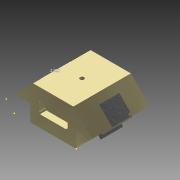
# Autodesk Inventor part: Correct middle piece Thursday 16
Saved by Autodesk Inventor 2015 (Build 190159000, 159)
## iProperties
Created: 2015-04-16
Part Number: Correct middle piece Thursday 16
Material: Generic
Document SubType Name: Modeling
Designer: Simrun
Density: 1 g/cm^3
Appearance: Gold - Metal
Author: Simrun
Autodesk Inventor part; units mm, degrees
sketch "Sketch1" plane through (0, 0, 0) normal (0, 0, 1) x (1, 0, 0)
  line L0 (0, 0) -> (171.45, 0)
  line L1 (171.45, 0) -> (171.45, 77.724)
  line L2 (171.45, 77.724) -> (0, 77.724)
  line L3 (0, 77.724) -> (0, 0)
  dimension "d0" = 171.45
  dimension "d1" = 77.724
  constraints: 8 end point, 2 parallel, 1 horizontal, 1 perpendicular
  measures "d0" distance of L2.end L1.end
  measures "d1" distance of L1.end L0.end
extrude "Extrusion1" add sketch "Sketch1" against normal blind 127
chamfer "Chamfer1" distance 41.275 angle 45 1 edges at (171.45, 77.724, -63.5)
chamfer "Chamfer2" distance 36.449 angle 45 1 edges at (171.45, 0, -63.5)
chamfer "Chamfer3" distance 41.275 angle 45 1 edges at (0, 77.724, -63.5)
chamfer "Chamfer4" distance 36.449 angle 45 1 edges at (0, 0, -63.5)
sketch "Sketch2" plane through (0, 0, 0) normal (0, 0, 1) x (1, 0, 0)
  point P0 (0, 0)
ref_plane "Work Plane1" through (0, 38.862, 0) normal (0, 1, 0) x (-1, 0, 0)
ref_plane "Work Plane4" through (85.725, 793.6029, -127) normal (1, 0, 0) x (0, 0, -1)
ref_plane "Work Plane2" through (130.175, 77.724, -127) normal (0.9980779, 0.0619722, 0) x (0, 0, 1)
ref_plane "Work Plane3" through (41.275, 77.724, -127) normal (0.9980779, -0.0619722, 0) x (0, 0, 1)
ref_plane "Work Plane5" through (171.45, 36.449, 0) normal (0, 1, 0) x (0, 0, -1)
ref_plane "Work Plane7" through (136.398, 36.449, 0) normal (1, 0, 0) x (0, 1, 0)
ref_plane "Work Plane6" through (171.45, 36.449, 0) normal (1, 0, 0) x (0, 1, 0)
sketch "Sketch3" plane through (136.398, 36.449, 0) normal (1, 0, 0) x (0, 1, 0)
  line L0 (-36.449, 0) -> (0, 0)
  line L1 (0, 0) -> (41.275, 0) projected
  arc A0 (-34.925, -22.225) -> (0, 0) centre (-33.1023, 13.4644) ccw
  line L2 (-34.925, -22.225) -> (-34.925, 0)
  dimension "d17" = 36.449
  constraints: 4 end point, 2 point on circle, 2 point on line, 1 centre point, 1 vertical
  measures "d17" distance of L0.start L0.end
extrude "Extrusion2" add sketch "Sketch3" along normal blind 34.925
sketch "Sketch4" plane through (171.323, 36.449, 0) normal (1, 0, 0) x (0, 0, -1)
  line L0 (0, -34.925) -> (0, 0)
  line L1 (0, -36.449) -> (0, 0) projected
  arc A0 (22.225, -34.925) -> (0, 0) centre (-13.4644, -33.1023) ccw
  line L2 (22.225, -34.925) -> (0, -34.925)
  line L3 (127, -36.449) -> (0, -36.449) projected
  constraints: 4 end point, 2 point on circle, 1 centre point, 1 collinear, 1 parallel
extrude "Extrusion3" cut sketch "Sketch4" against normal blind 34.925
mirror "Mirror1" about plane through (85.725, 793.6029, -127) normal (1, 0, 0) of "Extrusion3"
sketch "Sketch5" plane through (130.175, 77.724, -127) normal (0.7071068, 0.7071068, 0) x (-0.7071068, 0.7071068, 0)
  line L0 (-58.3717, 127) -> (-58.3717, 0) projected
  line L1 (-58.3717, 84.1375) -> (-17.4625, 84.1375)
  line L2 (-17.4625, 84.1375) -> (-17.4625, 39.6875)
  line L3 (-17.4625, 39.6875) -> (-58.3717, 39.6875)
  line L4 (-58.3717, 39.6875) -> (-58.3717, 84.1375)
  point P0 (37.0885, 127)
  constraints: 8 end point, 2 parallel, 1 horizontal, 1 perpendicular, 1 point on line
extrude "Extrusion4" add sketch "Sketch5" along normal blind 2.54
sketch "Sketch6" plane through (135.001, 0, 0) normal (0.7071068, -0.7071068, 0) x (-0.7071068, -0.7071068, 0)
  line L0 (-51.5467, 42.8625) -> (-20.6375, 42.8625)
  line L1 (-20.6375, 42.8625) -> (-20.6375, 87.3125)
  line L2 (-20.6375, 87.3125) -> (-51.5467, 87.3125)
  line L3 (-51.5467, 87.3125) -> (-51.5467, 42.8625)
  point P0 (95.4601, 0)
  constraints: 8 end point, 2 parallel, 1 horizontal, 1 perpendicular
extrude "Extrusion5" add sketch "Sketch6" along normal blind 2.54
sketch "Sketch7" plane through (135.001, 0, 0) normal (0.7071068, -0.7071068, 0) x (-0.7071068, -0.7071068, 0)
  line L0 (-17.4625, 42.8625) -> (-10.4467, 42.8625)
  line L1 (-10.4467, 42.8625) -> (-10.4467, 87.3125)
  line L2 (-10.4467, 87.3125) -> (-17.4625, 87.3125)
  line L3 (-17.4625, 87.3125) -> (-17.4625, 42.8625)
  point P0 (95.4601, 0)
  constraints: 8 end point, 2 parallel, 1 horizontal, 1 perpendicular
extrude "Extrusion6" add sketch "Sketch7" along normal blind 7.62
sketch "Sketch8" plane through (131.9711, 79.5201, -127) normal (0.7071068, 0.7071068, 0) x (0, 0, 1)
  line L0 (46.0375, 52.3875) -> (41.275, 52.3875)
  line L1 (41.275, 52.3875) -> (41.275, 57.15)
  line L2 (41.275, 57.15) -> (46.0375, 57.15)
  line L3 (46.0375, 57.15) -> (46.0375, 52.3875)
  point P0 (127, -37.0885)
  constraints: 8 end point, 2 parallel, 1 horizontal, 1 perpendicular
extrude "Extrusion7" add sketch "Sketch8" along normal blind 2.54
sketch "Sketch9" plane through (136.398, 36.449, 0) normal (1, 0, 0) x (0, 0, -1)
  point P0 (0, -36.449)
ref_plane "Work Plane10" through (130.175, 77.724, -63.5) normal (0, 0, 1) x (-1, 0, 0)
ref_plane "Work Plane8" through (130.175, 77.724, -127) normal (0, 0, 1) x (-1, 0, 0)
ref_plane "Work Plane9" through (41.275, 77.724, 0) normal (0, 0, -1) x (1, 0, 0)
mirror "Mirror2" about plane through (130.175, 77.724, -63.5) normal (0, 0, 1) of "Extrusion3"
mirror "Mirror3" about plane through (130.175, 77.724, -63.5) normal (0, 0, 1) of "Extrusion3", "Mirror1"
sketch "Sketch10" plane through (130.175, 77.724, 0) normal (0, 1, 0) x (1, 0, 0)
  line L0 (-88.9, 0) -> (-88.9, 127) projected
  line L1 (-88.9, 63.5) -> (0, 63.5)
  line L2 (0, 127) -> (0, 0) projected
  line L3 (4.826, 127) -> (-93.726, 127) projected
  line L4 (-44.45, 127) -> (-44.45, 0)
  line L5 (-93.726, 0) -> (4.826, 0) projected
  circle A0 centre (-44.45, 63.5) radius 4.572
  point P0 (-130.175, 0)
  dimension "d30" = 9.144
  constraints: 5 midpoint, 4 end point, 1 centre point
  measures "d30" diameter of A0
extrude "Extrusion8" cut sketch "Sketch10" against normal blind 10.16 contours A0 L4 L1 | L1 L4 A0 | L4 L1 A0 | L4 A0 L1
sketch "Sketch11" plane through (136.398, 36.449, 0) normal (1, 0, 0) x (0, 0, -1)
  point P0 (0, -36.449)
sketch "Sketch12" plane through (136.398, 1.524, -127) normal (1, 0, 0) x (0, 0, -1)
  point P0 (-127, -1.524)
sketch "Sketch13" plane through (0, 0, 0) normal (0, 0, 1) x (1, 0, 0)
  line L0 (53.975, 51.562) -> (53.975, 26.162)
  line L1 (53.975, 51.562) -> (117.475, 51.562)
  line L2 (53.975, 26.162) -> (117.475, 26.162)
  line L3 (117.475, 26.162) -> (117.475, 51.562)
  line L4 (136.398, 1.524) -> (136.398, 36.449) projected
  line L5 (130.175, 77.724) -> (41.275, 77.724) projected
  point P0 (0, 0)
  dimension "d33" = 25.4
  dimension "d34" = 63.5
  dimension "d35" = 18.923
  dimension "d36" = 26.162
  constraints: 8 end point, 2 horizontal, 1 perpendicular, 1 vertical
  measures "d33" distance of L0.start L0.end
  measures "d34" distance of L0.start L1.end
  measures "d35" distance between parallel lines of L3 L4
  measures "d36" distance between parallel lines of L5 L1
extrude "Extrusion9" cut sketch "Sketch13" against normal blind 14.478
fillet "Fillet1" radius 5.08 4 edges at (53.975, 26.162, -7.239) (53.975, 51.562, -7.239) (117.475, 51.562, -7.239) (117.475, 26.162, -7.239)
sketch "Sketch14" plane through (0, 0, -127) normal (0, 0, -1) x (-1, 0, 0)
  line L0 (-116.205, 50.673) -> (-55.245, 50.673)
  line L1 (-55.245, 50.673) -> (-55.245, 27.051)
  line L2 (-59.055, 51.562) -> (-112.395, 51.562) projected
  line L3 (-116.205, 50.673) -> (-116.205, 27.051)
  line L4 (-116.205, 27.051) -> (-55.245, 27.051)
  line L5 (-41.275, 77.724) -> (-130.175, 77.724) projected
  line L6 (-35.052, 1.524) -> (-35.052, 36.449) projected
  point P0 (0, 0)
  dimension "d40" = 60.96
  dimension "d41" = 23.622
  dimension "d42" = 27.051
  dimension "d43" = 20.193
  constraints: 8 end point, 2 perpendicular, 1 horizontal, 1 vertical
  measures "d40" distance of L0.start L0.end
  measures "d41" distance of L0.end L1.end
  measures "d42" distance between parallel lines of L5 L0
  measures "d43" distance between parallel lines of L6 L1
extrude "Extrusion10" cut sketch "Sketch14" against normal blind 14.478
fillet "Fillet2" radius 5.08 4 edges at (116.205, 50.673, -119.761) (55.245, 50.673, -119.761) (55.245, 27.051, -119.761) (116.205, 27.051, -119.761)
sketch "Sketch15" plane through (41.275, 77.724, -127) normal (-0.7071068, 0.7071068, 0) x (-0.7071068, -0.7071068, 0)
  line L0 (3.0559, 55.5567) -> (53.8559, 55.5567) construction
  line L1 (53.8559, 55.5567) -> (53.8559, 4.7567) construction
  line L2 (53.8559, 4.7567) -> (3.0559, 4.7567) construction
  line L3 (3.0559, 4.7567) -> (3.0559, 55.5567) construction
  point P0 (84.145, 127)
  dimension "d48" = 50.8
  constraints: 2 other
  measures "d48" distance of L0.end L1.end
body "Solid1"
